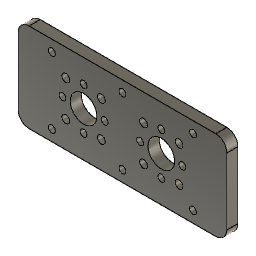
testBaseEncoder v1 (Autodesk Fusion 360 design; units mm, degrees)
Autodesk Fusion 360 part; units mm, degrees
sketch "Sketch1" plane through (0, 0, 0) normal (0, 1, 0) x (1, 0, 0)
  circle A0 centre (101.4766, 0) radius 9.5 construction
  circle A1 centre (136.4766, 0) radius 9.5 construction
  circle A2 centre (101.4766, 0) radius 16.5 construction
  circle A3 centre (136.4766, 0) radius 16.5 construction
  circle A4 centre (101.4766, -9.5) radius 1.55
  circle A5 centre (110.9766, 0) radius 1.55
  circle A6 centre (101.4766, 9.5) radius 1.55
  circle A7 centre (91.9766, 0) radius 1.55
  circle A8 centre (136.4766, -9.5) radius 1.55
  circle A9 centre (145.9766, 0) radius 1.55
  circle A10 centre (136.4766, 9.5) radius 1.55
  circle A11 centre (126.9766, 0) radius 1.55
  circle A12 centre (118.9766, -15) radius 1.55
  circle A13 centre (118.9766, 15) radius 1.55
  line L0 (91.9766, -20) -> (145.9766, -20)
  line L1 (145.9766, 20) -> (91.9766, 20)
  line L2 (91.9766, 0) -> (145.9766, 0) construction
  circle A14 centre (101.4766, 0) radius 6
  circle A15 centre (136.4766, 0) radius 6
  line L3 (76.9766, 20) -> (160.9766, 20)
  line L4 (165.9766, 15) -> (165.9766, -15)
  line L5 (160.9766, -20) -> (76.9766, -20)
  line L6 (71.9766, -15) -> (71.9766, 15)
  line L7 (71.9766, 20) -> (165.9766, -20) construction
  line L8 (165.9766, 20) -> (71.9766, -20) construction
  arc A16 (71.9766, -15) -> (76.9766, -20) centre (76.9766, -15) ccw
  arc A17 (76.9766, 20) -> (71.9766, 15) centre (76.9766, 15) ccw
  arc A18 (165.9766, 15) -> (160.9766, 20) centre (160.9766, 15) ccw
  arc A19 (160.9766, -20) -> (165.9766, -15) centre (160.9766, -15) ccw
  line L9 (93.4766, -8) -> (109.4766, -8) construction
  line L10 (109.4766, -8) -> (109.4766, 8) construction
  line L11 (109.4766, 8) -> (93.4766, 8) construction
  line L12 (93.4766, 8) -> (93.4766, -8) construction
  line L13 (93.4766, -8) -> (109.4766, 8) construction
  line L14 (109.4766, -8) -> (93.4766, 8) construction
  line L15 (128.4766, -8) -> (144.4766, -8) construction
  line L16 (144.4766, -8) -> (144.4766, 8) construction
  line L17 (144.4766, 8) -> (128.4766, 8) construction
  line L18 (128.4766, 8) -> (128.4766, -8) construction
  line L19 (128.4766, -8) -> (144.4766, 8) construction
  line L20 (144.4766, -8) -> (128.4766, 8) construction
  circle A20 centre (93.4766, -8) radius 1.75
  circle A21 centre (109.4766, -8) radius 1.75
  circle A22 centre (93.4766, 8) radius 1.75
  circle A23 centre (109.4766, 8) radius 1.75
  circle A24 centre (128.4766, -8) radius 1.75
  circle A25 centre (144.4766, -8) radius 1.75
  circle A26 centre (128.4766, 8) radius 1.75
  circle A27 centre (144.4766, 8) radius 1.75
  circle A28 centre (87.2266, -15) radius 1.55
  circle A29 centre (87.2266, 15) radius 1.55
  circle A30 centre (150.7266, -15) radius 1.55
  circle A31 centre (150.7266, 15) radius 1.55
  point P0 (101.4766, 0)
  point P1 (136.4766, 0)
  point P2 (118.9766, 0)
  point P3 (101.4766, 0)
  point P4 (136.4766, 0)
  point P5 (118.9766, 0)
  point P6 (101.4766, 0)
  point P7 (136.4766, 0)
  dimension "d1" = 19
  dimension "d3" = 33
  dimension "d4" = 33
  dimension "d6" = 35
  dimension "d7" = 3.1
  dimension "d9" = 360
  dimension "d10" = 3.1
  dimension "d12" = 360
  dimension "d17" = 17.5
  dimension "d18" = 3.1
  dimension "d19" = 3.1
  dimension "d24" = 12
  dimension "d25" = 12
  dimension "d38" = 94
  dimension "d39" = 40
  dimension "d40" = 5
  dimension "d45" = 16
  dimension "d46" = 16
  dimension "d47" = 16
  dimension "d48" = 16
  dimension "d49" = 3.5
  dimension "d50" = 3.5
  dimension "d51" = 3.5
  dimension "d52" = 3.5
  dimension "d53" = 3.5
  dimension "d54" = 3.5
  dimension "d55" = 3.5
  dimension "d56" = 3.5
  dimension "d57" = 3.1
  dimension "d58" = 3.1
  dimension "d59" = 3.1
  dimension "d60" = 3.1
  dimension "d61" = 15
  dimension "d62" = 15
  dimension "d63" = 15
  dimension "d64" = 15
  dimension "d65" = 31.75
  dimension "d66" = 31.75
  dimension "d67" = 31.75
  dimension "d68" = 31.75
  constraint horizontal P6 P7
  constraint coincident P6 P0
  constraint coincident P7 P1
  constraint coincident P6 P3
  constraint coincident P7 P4
  constraint coincident A0 A4.centre
  constraint coincident A1 A8.centre
  constraint parallel L0 L1
  constraint coincident A9.centre L2.end
  constraint horizontal L2
  constraint coincident A7.centre L2.start
  constraint concentric A2 A14
  constraint concentric A3 A15
  constraint horizontal L3
  constraint perpendicular L3 L4
  constraint parallel L3 L5
  constraint parallel L4 L6
  constraint coincident L7 P5
  constraint coincident L8 P5
  constraint coincident P5 P2
  constraint coincident L8.end L6
  constraint coincident L8.end L5
  constraint tangent L6 A16
  constraint tangent L5 A16
  constraint coincident L7.start L6
  constraint coincident L7.start L3
  constraint tangent L6 A17
  constraint tangent L3 A17
  constraint equal A16 A17
  constraint coincident L8.start L3
  constraint coincident L8.start L4
  constraint tangent L3 A18
  constraint tangent L4 A18
  constraint equal A16 A18
  constraint coincident L7.end L4
  constraint coincident L7.end L5
  constraint tangent L4 A19
  constraint tangent L5 A19
  constraint equal A16 A19
  constraint horizontal L9
  constraint perpendicular L9 L10
  constraint parallel L9 L11
  constraint parallel L10 L12
  constraint coincident L13 P6
  constraint coincident L14 P6
  constraint horizontal L15
  constraint perpendicular L15 L16
  constraint parallel L15 L17
  constraint parallel L16 L18
  constraint coincident L19 P7
  constraint coincident L20 P7
  constraint coincident L9.start L12.end
  constraint coincident L9.end L10.start
  constraint coincident L11.end L12.start
  constraint coincident L10.end L11.start
  constraint coincident L15.start L18.end
  constraint coincident L15.end L16.start
  constraint coincident L17.end L18.start
  constraint coincident L16.end L17.start
  measures "d1" diameter of A0
  measures "d3" diameter of A2
  measures "d4" diameter of A3
  measures "d6" distance of P0 P7
  measures "d7" diameter of A4
  measures "d10" diameter of A8
  measures "d17" distance of P6 P5
  measures "d18" diameter of A12
  measures "d19" diameter of A13
  measures "d24" diameter of A14
  measures "d25" diameter of A15
  measures "d38" distance of L7.end L8.end
  measures "d39" distance of L8.start L7.end
  measures "d40" radius of A16
  measures "d45" distance of L10.end L11.end
  measures "d46" distance of L9.end L10.end
  measures "d47" distance of L16.end L17.end
  measures "d48" distance of L15.end L16.end
  measures "d49" diameter of A20
  measures "d50" diameter of A21
  measures "d51" diameter of A22
  measures "d52" diameter of A23
  measures "d53" diameter of A24
  measures "d54" diameter of A25
  measures "d55" diameter of A26
  measures "d56" diameter of A27
  measures "d57" diameter of A28
  measures "d58" diameter of A29
  measures "d59" diameter of A30
  measures "d60" diameter of A31
  measures "d61" vertical distance of P5 A28.centre
  measures "d62" vertical distance of P5 A29.centre
  measures "d63" vertical distance of P5 A30.centre
  measures "d64" vertical distance of P5 A31.centre
  measures "d65" horizontal distance of P5 A28.centre
  measures "d66" horizontal distance of P5 A30.centre
  measures "d67" horizontal distance of P5 A31.centre
  measures "d68" horizontal distance of P5 A29.centre
extrude "Extrude1" add sketch "Sketch1" along normal blind 5
equation "d17 = d6 / 2"
equation "d49 = d54"
equation "d50 = d54"
equation "d51 = d54"
equation "d52 = d54"
equation "d53 = d54"
equation "d55 = d54"
equation "d56 = d54"
equation "d61 = d63"
equation "d62 = d63"
equation "d64 = d63"
equation "d66 = d65"
equation "d67 = d65"
equation "d68 = d65"
